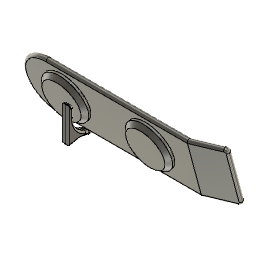
model (Autodesk Fusion 360 design; units mm, degrees)
Autodesk Fusion 360 part; units mm, degrees
sketch "Sketch1" plane through (0, 0, 0) normal (0, 0, 1) x (1, 0, 0) in component "board"
  line L0 (0, 0) -> (447, 0)
  line L1 (445.1645, 12) -> (0, 12)
  line L2 (0, 12) -> (0, 0)
  line L3 (447, 0) -> (530, 26)
  line L4 (530, 26) -> (526.4128, 37.4513)
  line L5 (526.4128, 37.4513) -> (445.1645, 12)
  line L6 (0, 0) -> (0, 50) construction
  line L7 (0, 50) -> (530, 50) construction
  line L8 (530, 50) -> (530, 26) construction
  dimension "d1" = 530
  dimension "d2" = 12
  dimension "d3" = 83
  dimension "d4" = 12
  dimension "d12" = 26
  dimension "d15" = 50
  constraint horizontal L0
  constraint horizontal L1
  constraint vertical L2
  constraint coincident L0.start L2.end
  constraint parallel L3 L5
  constraint perpendicular L4 L5
  constraint coincident L1.start L5.end
  constraint perpendicular L1 L6
  constraint perpendicular L6 L7
  constraint perpendicular L7 L8
  measures "d1" distance of L2 L3.end
  measures "d2" distance of L0.start L1.end
  measures "d3" horizontal distance of L0.end L3.end
  measures "d4" distance of L3.end L4.end
  measures "d12" vertical distance of L0.end L3.end
  measures "d15" distance of L0.start L7
extrude "Extrude1" add sketch "Sketch1" along normal blind 152 makes body 1 in component "board"
sketch "Sketch2" plane through (0, 0, 0) normal (0, -1, 0) x (1, 0, 0) in component "board"
  line L0 (0, 0) -> (447, 0)
  line L1 (447, 0) -> (447, 152)
  line L2 (447, 152) -> (0, 152)
  line L3 (0, 152) -> (0, 0)
  circle A0 centre (113.429, 76) radius 60
  circle A1 centre (333.571, 76) radius 60
  line L4 (113.429, 76) -> (333.571, 76) construction
  line L5 (113.429, 76) -> (0, 76) construction
  line L6 (333.571, 76) -> (447, 76) construction
  line L7 (223.5, 76) -> (223.5, 152) construction
  line L8 (223.5, 76) -> (223.5, 0) construction
  dimension "d22" = 120
  constraint coincident A0.centre L4.start
  constraint coincident A1.centre L4.end
  constraint horizontal L4
  constraint equal A0 A1
  constraint coincident L3 L5.end
  constraint perpendicular L3 L5
  constraint coincident L1 L6.end
  constraint perpendicular L1 L6
  constraint equal L5 L6
  constraint midpoint L4 L7.start
  constraint midpoint L2 L7.end
  constraint midpoint L0 L8.end
  constraint equal L7 L8
  measures "d22" diameter of A0
extrude "Extrude2" add sketch "Sketch2" along normal blind 16 contours A0 | A1 bodies 1 in component "board"
chamfer "Chamfer1" distance 10 angle 45 2 faces at (347.1329, -16, 94.4192) (107.8865, -16, 110.0713) on bodies 1 in component "board"
fillet "Fillet1" radius 76 2 edges at (0, 6, 152) (0, 6, 0) on bodies 1 in component "board"
fillet "Fillet2" radius 10 2 edges at (528.2064, 31.7257, 152) (528.2064, 31.7257, 0) on bodies 1 in component "board"
fillet "Fillet3" radius 6 6 faces at (0, 8, 75.9949) (322.7164, 4, 152) (522.4386, 32.0147, 150.8884) (528.8043, 29.8171, 54) (522.4386, 32.0147, 1.1116) (322.7164, 4, 0) on bodies 1 in component "board"
move_body "Move1" bodies 1 to x (1, 0, 0) y (0, 0.965926, 0.258819) z (0, -0.258819, 0.965926) at (0, 50, 0) in component "board"
sketch "Sketch1 (2)" plane through (0, 0, 0) normal (0, 1, 0) x (1, 0, 0) in component "wall"
  line L0 (-40, 70) -> (560, 70)
  line L1 (560, 70) -> (560, -230)
  line L2 (560, -230) -> (-40, -230)
  line L3 (-40, -230) -> (-40, 70)
  dimension "d16" = 600
  dimension "d17" = 300
  dimension "d18" = 40
  dimension "d19" = 70
  constraint horizontal L0
  constraint vertical L1
  constraint horizontal L2
  constraint vertical L3
  measures "d16" distance of L1.end L2.end
  measures "d17" distance of L0.end L1.end
  measures "d18" distance of L3 origin
  measures "d19" distance of origin L0
extrude "Extrude1'" add sketch "Sketch1 (2)" against normal blind 10 separate body makes body 2 in component "wall"
sketch "Sketch1 (3)" plane through (0, 0, 0) normal (1, 0, 0) x (0, 1, 0) in component "hook"
  line L0 (0, 230) -> (0, -70)
  line L1 (42.7884, 5.1575) -> (52.1772, 1.7152)
  line L2 (59.6805, 4.8128) -> (61.7936, 9.3443) construction
  line L3 (61.7936, 9.3443) -> (70.8567, 5.1181) construction
  line L4 (70.8567, 5.1181) -> (68.7436, 0.5866) construction
  line L5 (0, 81.7152) -> (0, -21.3777)
  line L6 (0, 230) -> (0, -70)
  arc A0 (52.1772, 1.7152) -> (59.6805, 4.8128) centre (54.2426, 7.3485) ccw
  arc A1 (50.6067, -8.2329) -> (68.7436, 0.5866) centre (54.2426, 7.3485) ccw
  line L7 (50.6067, -8.2329) -> (40.8683, -5.9605)
  arc A2 (48.4471, 5.7956) -> (60.0382, 8.9014) centre (54.2426, 7.3485) ccw
  arc A3 (10, 52.1017) -> (42.7884, 5.1575) centre (60, 52.1017) ccw
  arc A4 (40.8683, -5.9605) -> (15.5937, -6.6507) centre (29.5466, -54.4788) ccw
  line L8 (10, 52.1017) -> (10, 74.0229)
  line L9 (2.3077, 81.7152) -> (0, 81.7152)
  line L10 (1.5909, -8.6515) -> (0, -8.6515)
  arc A5 (68.7436, 0.5866) -> (59.6773, 4.8058) centre (64.212, 2.6997) ccw
  arc A6 (68.7436, 0.5866) -> (59.6805, 4.8128) centre (64.212, 2.6997) ccw
  line L11 (54.2426, 7.3485) -> (59.6805, 4.8128) construction
  arc A7 (10, 74.0229) -> (2.3077, 81.7152) centre (2.3077, 74.0229) ccw
  line L12 (10, -8.6515) -> (10.4353, -8.6515) construction
  line L13 (10.4353, -8.6515) -> (54.2426, -8.6515) construction
  arc A8 (1.5909, -8.6515) -> (15.5937, -6.6507) centre (1.5909, 41.3485) ccw
  dimension "d36" = 6
  dimension "d38" = 10
  dimension "d40" = 5
  dimension "d41" = 80
  dimension "d43" = 50
  dimension "d44" = 10
  dimension "d45" = 10
  dimension "d46" = 115
  dimension "d47" = 10
  dimension "d48" = 7.6923
  dimension "d49" = 7
  dimension "d50" = 50
  constraint coincident L0 L5.start
  constraint tangent L1 A0
  constraint tangent L2 A0
  constraint parallel L2 L4
  constraint perpendicular L2 L3
  constraint coincident A0.centre A1.centre
  constraint tangent L4 A1
  constraint tangent A1 L7
  constraint tangent A0 A2
  constraint tangent L1 A3
  constraint coincident L6 L5.end
  constraint tangent L7 A4
  constraint vertical L8
  constraint tangent A3 L8
  constraint perpendicular L8 L9
  constraint perpendicular L6 L10
  constraint coincident L6 L10.end
  constraint tangent L3 A5
  constraint tangent L4 A5
  constraint tangent L3 A6
  constraint tangent A2 A6
  constraint tangent L8 A7
  constraint tangent L9 A7
  constraint coincident A1 L13.end
  constraint tangent A1 L13
  constraint collinear L10 L13
  constraint equal L1 L7
  constraint coincident L12.start L10
  constraint coincident A4 L12.start
  constraint tangent L10 A8
  constraint tangent A4 A8
  measures "d36" radius of A0
  measures "d38" distance of L2.end L3.end
  measures "d40" distance of L3.end L4.end
  measures "d41" vertical distance of L5.start L1.end
  measures "d43" radius of A3
  measures "d44" distance of L6 L8
  measures "d45" distance of L12.start L10.end
  measures "d46" angle of L6 L11
  measures "d47" distance of L1.end L1.start
  measures "d48" radius of A7
  measures "d49" angle of L1 L7
  measures "d50" radius of A8
extrude "Extrude1''" add sketch "Sketch1 (3)" along normal blind 20 separate body makes body 3 in component "hook"
fillet "Fillet1'" radius 5 24 edges at (0, 1.1538, 81.7152) (0, 7.747, 79.4621) (0, 10, 63.0623) (0, 19.0087, 23.4711) (0, 47.4828, 3.4363) (0, 56.5322, 1.8025) (0, 66.3251, 7.2312) (0, 61.2396, -7.0405) (0, 45.7375, -7.0967) (0, 28.1865, -4.6756) (0, 8.6634, -8.1488) (0, 0.7955, -8.6515) (20, 0.7955, -8.6515) (20, 8.6634, -8.1488) (20, 28.1865, -4.6756) (20, 45.7375, -7.0967) (20, 61.2396, -7.0405) (20, 66.3251, 7.2312) (20, 56.5322, 1.8025) (20, 47.4828, 3.4363) (20, 19.0087, 23.4711) (20, 10, 63.0623) (20, 7.747, 79.4621) (20, 1.1538, 81.7152) on bodies 3 in component "hook"
sketch "Sketch2 (2)" plane through (0, 0, 0) normal (0, -1, 0) x (1, 0, 0) in component "hook"
  arc A0 (15, -8.6515) -> (20, -3.6515) centre (15, -3.6515) ccw
  line L0 (20, -3.6515) -> (20, 76.7152)
  arc A1 (20, 76.7152) -> (15, 81.7152) centre (15, 76.7152) ccw
  line L1 (15, 81.7152) -> (5, 81.7152)
  arc A2 (5, 81.7152) -> (0, 76.7152) centre (5, 76.7152) ccw
  line L2 (0, 76.7152) -> (0, -3.6515)
  arc A3 (0, -3.6515) -> (5, -8.6515) centre (5, -3.6515) ccw
  line L3 (5, -8.6515) -> (15, -8.6515)
  line L4 (0.7351, 76.1813) -> (19.4351, 76.1813)
  line L5 (19.4351, 76.1813) -> (19.4351, 6.3771)
  line L6 (9.9834, -2.9729) -> (9.9834, -2.9729)
  line L7 (0.7351, 6.3771) -> (0.7351, 76.1813)
  arc A4 (0.7351, 6.3771) -> (10.0851, -2.9729) centre (10.0851, 6.3771) ccw
  arc A5 (10.0851, -2.9729) -> (19.4351, 6.3771) centre (10.0851, 6.3771) ccw
  point P0 (0.7351, -11.8187)
  dimension "d58" = 18.7
  dimension "d59" = 88
  dimension "d60" = 9.35
  constraint horizontal L4
  constraint vertical L5
  constraint vertical L7
  constraint coincident P0 L7
  constraint tangent L7 A4
  constraint tangent L5 A5
  constraint equal A4 A5
  measures "d58" distance of L4.start L4.end
  measures "d59" distance of L4.start P0
  measures "d60" radius of A4
ref_plane "WorkPlane1" through (10, 25.8715, 36.5318) normal (-1, 0, 0) x (0, -1, 0) in component "hook"
split "Split1" by plane through (10, 25.8715, 36.5318) normal (-1, 0, 0) bodies 3 makes body 4 at (0, 10.5389, 12.5697) in component "hook"
component "hook" placed x (1, 0, 0) y (0, 1, 0) z (0, 0, 1) at (130, 0, 0)
component "board" placed x (1, 0, 0) y (0, 1, 0) z (0, 0, 1) at (0, 0, 0)
component "wall" placed x (1, 0, 0) y (0, 1, 0) z (0, 0, 1) at (0, 0, 0)
equation "d1 = height"
equation "d2 = thickness"
equation "d3 = aLength"
equation "d4 = d2"
equation "widht = 152 mm"
equation "height = 530 mm"
equation "thickness = 12 mm"
equation "projection = 16 mm"
equation "aLength = 83 mm"
equation "aProjection = 42 mm - projection"
equation "hookDepth = 50 mm"
equation "d12 = aProjection"
equation "d13 = widht"
equation "d15 = hookDepth"
equation "d24 = projection"
equation "d28 = widht / 2"
equation "d32 = thickness / 2"
equation "d36 = thickness / 2"
equation "hookThickness = 10 mm"
equation "d38 = hookThickness"
equation "d40 = hookThickness / 2"
equation "d41 = hookHeight"
equation "hookHeight = 80 mm"
equation "d44 = hookThickness"
equation "d45 = hookThickness"
equation "d47 = hookThickness"
equation "d48 = hookThickness / 1.3"
equation "d50 = 5 * hookThickness"
equation "hookWidth = 20 mm"
equation "d52 = hookWidth"
equation "d55 = hookThickness / 2"
equation "stripWidth = 18.7 mm"
equation "stripHeight = 88 mm"
equation "d58 = stripWidth"
equation "d59 = stripHeight"
equation "d60 = stripWidth / 2"
